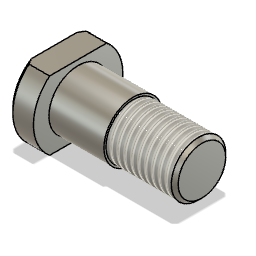
chamber bolts v3 (Autodesk Fusion 360 design; units mm, degrees)
Autodesk Fusion 360 part; units mm, degrees
sketch "Sketch1" plane through (0, 0, 0) normal (0, 0, 1) x (1, 0, 0)
  line L0 (0, 0) -> (0, 13)
  line L1 (0, 13) -> (7, 13)
  line L2 (7, 13) -> (7, 8.5)
  line L3 (7, 8.5) -> (23, 8.5)
  line L4 (23, 8.5) -> (23, 8)
  line L5 (23, 8) -> (43, 8)
  line L6 (43, 8) -> (43, 0)
  line L7 (43, 0) -> (0, 0)
  dimension "d1" = 7
  dimension "d3" = 16
  dimension "d4" = 20
  dimension "d5" = 13
  dimension "d6" = 8.5
  dimension "d7" = 8
  dimension "d8" = 43
  constraint vertical L0
  constraint perpendicular L0 L1
  constraint perpendicular L1 L2
  constraint perpendicular L2 L3
  constraint perpendicular L3 L4
  constraint perpendicular L4 L5
  constraint perpendicular L5 L6
  constraint perpendicular L0 L7
  constraint coincident L0.start L7.end
  measures "d1" distance of L0.end L1.end
  measures "d3" distance of L2.end L3.end
  measures "d4" distance of L4.end L5.end
  measures "d5" distance of L1 L7
  measures "d6" distance of L3 L7
  measures "d7" distance of L5 L7
  measures "d8" distance of L0.start L6.end
revolve "Revolve1" add sketch "Sketch1" angle 360 about axis through (43, 0, 0) along (-1, 0, 0)
thread "Thread1" "ISO Metric profile 16.0 M16x2 6g" major diameter 15.822 minor diameter 13.534 pitch 2 angle 60 resizes the face on face at (36.3333, 7.9602, 0.7965)
sketch "Sketch3" plane through (0, 0, 0) normal (1, 0, 0) x (0, 0, -1)
  circle A0 centre (0, 0) radius 13
  line L0 (8.3066, 10) -> (-8.3066, 10)
  line L1 (-8.3066, -10) -> (8.3066, -10)
  line L2 (-1.75, 0) -> (-22.5, 0)
  dimension "d11" = 20
  constraint coincident A0 L0.start
  constraint coincident A0 L0.end
  constraint horizontal L0
  constraint coincident A0 L1.start
  constraint coincident A0 L1.end
  constraint parallel L0 L1
  constraint symmetric L0 L1 L2
  measures "d11" distance of L0 L1
chamfer "Chamfer1" distance 1 angle 45 2 edges at (0, -4.701, 12.1203) (43, -7.3756, -2.8607)
extrude "Extrude1" cut sketch "Sketch3" along normal through all contours A0 L0 | A0 L1
equation "d6 = ( 17 / 2 ) * 1 mm"
